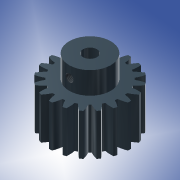
# Autodesk Inventor part: Spur Gear2
Saved by Autodesk Inventor 2017 SP1 (Build 210196100, 196)
## iProperties
Created: 2017-06-08
Part Number: Spur Gear2
Material: ABS Plastic
Document SubType Name: Modeling
Designer: zallen
Categories: <?xml version="1.0" encoding="UTF-16"?> <MemberInstance><Categories><FamilyTemplate><FamilyTemplateParameter ValueType="xs:double" Id="1" ObjectReferenceKey="da_z" ObjectType="kUserParameterObject"/><FamilyTemplateParameter ValueType="xs:double" Id="2" ObjectReferenceKey="da_b" ObjectType="kUserParameterObject"/><FamilyTemplateParameter ValueType="xs:double" Id="3" ObjectReferenceKey="da_beta" ObjectType="kUserParameterObject"/><FamilyTemplateParameter ValueType="xs:double" Id="4" ObjectReferenceKey="da_da" ObjectType="kUserParameterObject"/><FamilyTemplateParameter ValueType="xs:double" Id="5" ObjectReferenceKey="da_aw" ObjectType="kUserParameterObject"/><FamilyTemplateParameter ValueType="xs:string" Id="6" ObjectReferenceKey="EAIAABAAAACIAQAAAAAAAIAAAAAAAAAA" ObjectType="83910656" SubObjectId="SurfaceGeometry"/></FamilyTemplate><ParamToTemplateMap><ParamToTemplate CategoryParameter="//CategoryParameter[@InternalName='046C89C9-8512-4d59-83FE-43B91F4F132A']" TemplateParameter="1"/><ParamToTemplate CategoryParameter="//CategoryParameter[@InternalName='2552DF32-E462-4b46-AEBF-C6C7768E72AC']" TemplateParameter="2"/><ParamToTemplate CategoryParameter="//CategoryParameter[@InternalName='C9EE641D-15FC-4fae-A226-E94C4372FDD7']" TemplateParameter="3"/><ParamToTemplate><ParamToTemplate CategoryParameter="//CategoryParameter[@InternalName='00B6519A-459B-49c7-AD84-2E56D39A5744']" ConstantValue="0.000000"/></ParamToTemplate><ParamToTemplate><ParamToTemplate CategoryParameter="//CategoryParameter[@InternalName='04B31F0E-C7A6-4894-AA32-9629BEFACF47']" ConstantValue="1.000000"/></ParamToTemplate><ParamToTemplate><ParamToTemplate CategoryParameter="//CategoryParameter[@InternalName='43CBEC2E-7847-49e7-A936-2F7889FCB2D9']" ConstantValue="0.250000"/></ParamToTemplate><ParamToTemplate><ParamToTemplate CategoryParameter="//CategoryParameter[@InternalName='B1EFC894-105D-4ebd-86BF-FA20ED196853']" ConstantValue="0.350000"/></ParamToTemplate><ParamToTemplate><ParamToTemplate CategoryParameter="//CategoryParameter[@InternalName='51175063-3D10-4879-93E8-6246FE8B403D']" ConstantValue="2060000000.000000"/></ParamToTemplate><ParamToTemplate><ParamToTemplate CategoryParameter="//CategoryParameter[@InternalName='A3A52E27-4454-46a9-B0BD-C932399B70AF']" ConstantValue="0.300000"/></ParamToTemplate><ParamToTemplate><ParamToTemplate CategoryParameter="//CategoryParameter[@InternalName='91B76062-C214-41d9-B1B9-14D2AB99603D']" ConstantValue="0.130000"/></ParamToTemplate><ParamToTemplate><ParamToTemplate CategoryParameter="//CategoryParameter[@InternalName='374E806E-8B8A-4dda-A9AA-1039D6500AD2']" ConstantValue="7.692308"/></ParamToTemplate><ParamToTemplate><ParamToTemplate CategoryParameter="//CategoryParameter[@InternalName='2D373A89-B862-43d6-8D0B-0CBF12AB9F6C']" ConstantValue="0.349066"/></ParamToTemplate><ParamToTemplate CategoryParameter="//CategoryParameter[@InternalName='37777632-D6A2-4fac-9D53-DB8ACD95C989']" TemplateParameter="4"/><ParamToTemplate CategoryParameter="//CategoryParameter[@InternalName='FD1017F1-B727-4f7e-9707-0F86F1FF9423']" TemplateParameter="5"/><ParamToTemplate><ParamToTemplate CategoryParameter="//CategoryParameter[@InternalName='9E1B4470-B2D3-4ff1-B813-535BB4CDF51A']" ConstantValue="3520000.000000"/></ParamToTemplate><ParamToTemplate><ParamToTemplate CategoryParameter="//CategoryParameter[@InternalName='F8452263-BFF6-458c-9FB1-07C4B99E95CD']" ConstantValue="11400000.000000"/></ParamToTemplate><ParamToTemplate><ParamToTemplate CategoryParameter="//CategoryParameter[@InternalName='3E3BB259-FD49-497f-8171-6EBC954A3479']" ConstantValue="2.000000"/></ParamToTemplate><ParamToTemplate CategoryParameter="//CategoryParameter[@InternalName='27C3BAF2-7550-4e4b-AE2C-0DB134B7D9B7']" TemplateParameter="6"/></ParamToTemplateMap><Category DisplayName="Gear" InternalName="DC85795E-93AB-48d5-8EEE-5A27447B64BD" Mnemonic="Gear"><CategoryParameter DisplayName="z" InternalName="046C89C9-8512-4d59-83FE-43B91F4F132A" Mnemonic="z"/><CategoryParameter DisplayName="b" InternalName="2552DF32-E462-4b46-AEBF-C6C7768E72AC" Mnemonic="b"/><CategoryParameter DisplayName="||b|" InternalName="C9EE641D-15FC-4fae-A226-E94C4372FDD7" Mnemonic="beta"/><CategoryParameter DisplayName="x" InternalName="00B6519A-459B-49c7-AD84-2E56D39A5744" Mnemonic="x"/><CategoryParameter DisplayName="a*" InternalName="04B31F0E-C7A6-4894-AA32-9629BEFACF47" Mnemonic="a"/><CategoryParameter DisplayName="c*" InternalName="43CBEC2E-7847-49e7-A936-2F7889FCB2D9" Mnemonic="c"/><CategoryParameter DisplayName="r|.f|*" InternalName="B1EFC894-105D-4ebd-86BF-FA20ED196853" Mnemonic="rf"/><CategoryParameter DisplayName="E" InternalName="51175063-3D10-4879-93E8-6246FE8B403D" Mnemonic="E"/><CategoryParameter DisplayName="||m|" InternalName="A3A52E27-4454-46a9-B0BD-C932399B70AF" Mnemonic="mi"/><Category DisplayName="SpurGear" InternalName="26C5A22E-A91E-4dfd-A3B3-23CCAFAE1764" Mnemonic="SpurGear"><CategoryParameter DisplayName="m" InternalName="91B76062-C214-41d9-B1B9-14D2AB99603D" Mnemonic="m"/><CategoryParameter DisplayName="P" InternalName="374E806E-8B8A-4dda-A9AA-1039D6500AD2" Mnemonic="PP"/><CategoryParameter DisplayName="||a|" InternalName="2D373A89-B862-43d6-8D0B-0CBF12AB9F6C" Mnemonic="alpha"/><CategoryParameter DisplayName="d|.a|" InternalName="37777632-D6A2-4fac-9D53-DB8ACD95C989" Mnemonic="da"/><CategoryParameter DisplayName="a|.w|" InternalName="FD1017F1-B727-4f7e-9707-0F86F1FF9423" Mnemonic="aw"/><CategoryParameter DisplayName="||s||.Flim|" InternalName="9E1B4470-B2D3-4ff1-B813-535BB4CDF51A" Mnemonic="sFlim"/><CategoryParameter DisplayName="||s||.Hlim|" InternalName="F8452263-BFF6-458c-9FB1-07C4B99E95CD" Mnemonic="sHlim"/><CategoryParameter DisplayName="type" InternalName="3E3BB259-FD49-497f-8171-6EBC954A3479" Mnemonic="type"/><CategoryParameter DisplayName="PitchDiameter" InternalName="27C3BAF2-7550-4e4b-AE2C-0DB134B7D9B7" Mnemonic="IDS_PITCHDIAM"/></Category></Category></Categories></MemberInstance>
Density: 1.06 g/cm^3
Appearance: CR Dark Blue
CustomPartVersion: 1
Author: zallen
Autodesk Inventor part; units mm, degrees
sketch "Sketch1" plane through (0, 0, 0) normal (0, 0, 1) x (1, 0, 0)
  circle A0 centre (0, 0) radius 14.3
  dimension "d0" = 28.6
  constraints: 1 centre point
  measures "d0" diameter of A0
extrude "Extrusion1" add sketch "Sketch1" along normal blind 15
ref_plane "Work Plane2" through (0, 0, 7.5) normal (0, 0, 1) x (1, 0, 0)
sketch "Sketch2" plane through (0, 0, 0) normal (0, 0, -1) x (-1, 0, 0)
  circle A0 centre (0, 0) radius 14.3 projected
  circle A1 centre (0, 0) radius 13
  dimension "d3" = 26
  constraints: 1 centre point, 1 coincident
  measures "d3" diameter of A1
surface extrude "Pitch Diameter" sketch "Sketch2" against normal through all shown no curves A1
ref_plane "Work Plane8" through (0, 0, 0) normal (0.9876883, 0.1564345, 0) x (0, 0, 1)
ref_plane "Work Plane9" through (0, 0, 0) normal (1, 0, 0) x (0, 1, 0)
spur gear teeth "Spur Gear" teeth 20 pitch diameter 26 tip diameter 28.6 root diameter 22.75 face width 15 start plane through (0, 0, 0) normal (0, 0, -1) x (-1, 0, 0)
sketch "Sketch3" plane through (0, 0, 15) normal (0, 0, 1) x (1, 0, 0)
  circle A0 centre (0, 0) radius 2.5
  dimension "d49" = 5
  constraints: 1 centre point, 1 coincident
  measures "d49" diameter of A0
extrude "Extrusion2" cut sketch "Sketch3" against normal through all
sketch "Sketch4" plane through (0, 0, 15) normal (0, 0, 1) x (1, 0, 0)
  circle A0 centre (0, 0) radius 7.5
  circle A1 centre (0, 0) radius 2.5
  circle A2 centre (0, 0) radius 2.5 projected
  arc A3 (-4.9495, 13.4161) -> (-4.7623, 10.3301) centre (5.7891, 12.5189) ccw projected
  arc A4 (-4.7623, 10.3301) -> (-5.5581, 9.9246) centre (0, 0) ccw projected
  arc A5 (-5.5581, 9.9246) -> (-7.9447, 11.89) centre (-13.5308, 2.6749) ccw projected
  arc A6 (-7.9447, 11.89) -> (-8.853, 11.23) centre (0, 0) ccw projected
  arc A7 (-8.853, 11.23) -> (-7.7214, 8.3529) centre (1.6372, 13.6952) ccw projected
  arc A8 (-7.7214, 8.3529) -> (-8.3529, 7.7214) centre (0, 0) ccw projected
  arc A9 (-8.3529, 7.7214) -> (-11.23, 8.853) centre (-13.6952, -1.6372) ccw projected
  arc A10 (-11.23, 8.853) -> (-11.89, 7.9447) centre (0, 0) ccw projected
  arc A11 (-11.89, 7.9447) -> (-9.9246, 5.5581) centre (-2.6749, 13.5308) ccw projected
  arc A12 (-9.9246, 5.5581) -> (-10.3301, 4.7623) centre (0, 0) ccw projected
  arc A13 (-10.3301, 4.7623) -> (-13.4161, 4.9495) centre (-12.5189, -5.7891) ccw projected
  arc A14 (-13.4161, 4.9495) -> (-13.7631, 3.8816) centre (0, 0) ccw projected
  arc A15 (-13.7631, 3.8816) -> (-11.1564, 2.2192) centre (-6.7253, 12.042) ccw projected
  arc A16 (-11.1564, 2.2192) -> (-11.2962, 1.337) centre (0, 0) ccw projected
  arc A17 (-11.2962, 1.337) -> (-14.289, 0.5614) centre (-10.1173, -9.3744) ccw projected
  arc A18 (-14.289, 0.5614) -> (-14.289, -0.5614) centre (0, 0) ccw projected
  arc A19 (-14.289, -0.5614) -> (-11.2962, -1.337) centre (-10.1173, 9.3744) ccw projected
  arc A20 (-11.2962, -1.337) -> (-11.1564, -2.2192) centre (0, 0) ccw projected
  arc A21 (-11.1564, -2.2192) -> (-13.7631, -3.8816) centre (-6.7253, -12.042) ccw projected
  arc A22 (-13.7631, -3.8816) -> (-13.4161, -4.9495) centre (0, 0) ccw projected
  arc A23 (-13.4161, -4.9495) -> (-10.3301, -4.7623) centre (-12.5189, 5.7891) ccw projected
  arc A24 (-10.3301, -4.7623) -> (-9.9246, -5.5581) centre (0, 0) ccw projected
  arc A25 (-9.9246, -5.5581) -> (-11.89, -7.9447) centre (-2.6749, -13.5308) ccw projected
  arc A26 (-11.89, -7.9447) -> (-11.23, -8.853) centre (0, 0) ccw projected
  arc A27 (-11.23, -8.853) -> (-8.3529, -7.7214) centre (-13.6952, 1.6372) ccw projected
  arc A28 (-8.3529, -7.7214) -> (-7.7214, -8.3529) centre (0, 0) ccw projected
  arc A29 (-7.7214, -8.3529) -> (-8.853, -11.23) centre (1.6372, -13.6952) ccw projected
  arc A30 (-8.853, -11.23) -> (-7.9447, -11.89) centre (0, 0) ccw projected
  arc A31 (-7.9447, -11.89) -> (-5.5581, -9.9246) centre (-13.5308, -2.6749) ccw projected
  arc A32 (-5.5581, -9.9246) -> (-4.7623, -10.3301) centre (0, 0) ccw projected
  arc A33 (-4.7623, -10.3301) -> (-4.9495, -13.4161) centre (5.7891, -12.5189) ccw projected
  arc A34 (-4.9495, -13.4161) -> (-3.8816, -13.7631) centre (0, 0) ccw projected
  arc A35 (-3.8816, -13.7631) -> (-2.2192, -11.1564) centre (-12.042, -6.7253) ccw projected
  arc A36 (-2.2192, -11.1564) -> (-1.337, -11.2962) centre (0, 0) ccw projected
  arc A37 (-1.337, -11.2962) -> (-0.5614, -14.289) centre (9.3744, -10.1173) ccw projected
  arc A38 (-0.5614, -14.289) -> (0.5614, -14.289) centre (0, 0) ccw projected
  arc A39 (0.5614, -14.289) -> (1.337, -11.2962) centre (-9.3744, -10.1173) ccw projected
  arc A40 (1.337, -11.2962) -> (2.2192, -11.1564) centre (0, 0) ccw projected
  arc A41 (2.2192, -11.1564) -> (3.8816, -13.7631) centre (12.042, -6.7253) ccw projected
  arc A42 (3.8816, -13.7631) -> (4.9495, -13.4161) centre (0, 0) ccw projected
  arc A43 (4.9495, -13.4161) -> (4.7623, -10.3301) centre (-5.7891, -12.5189) ccw projected
  arc A44 (4.7623, -10.3301) -> (5.5581, -9.9246) centre (0, 0) ccw projected
  arc A45 (5.5581, -9.9246) -> (7.9447, -11.89) centre (13.5308, -2.6749) ccw projected
  arc A46 (7.9447, -11.89) -> (8.853, -11.23) centre (0, 0) ccw projected
  arc A47 (8.853, -11.23) -> (7.7214, -8.3529) centre (-1.6372, -13.6952) ccw projected
  arc A48 (7.7214, -8.3529) -> (8.3529, -7.7214) centre (0, 0) ccw projected
  arc A49 (8.3529, -7.7214) -> (11.23, -8.853) centre (13.6952, 1.6372) ccw projected
  arc A50 (11.23, -8.853) -> (11.89, -7.9447) centre (0, 0) ccw projected
  arc A51 (11.89, -7.9447) -> (9.9246, -5.5581) centre (2.6749, -13.5308) ccw projected
  arc A52 (9.9246, -5.5581) -> (10.3301, -4.7623) centre (0, 0) ccw projected
  arc A53 (10.3301, -4.7623) -> (13.4161, -4.9495) centre (12.5189, 5.7891) ccw projected
  arc A54 (13.4161, -4.9495) -> (13.7631, -3.8816) centre (0, 0) ccw projected
  arc A55 (13.7631, -3.8816) -> (11.1564, -2.2192) centre (6.7253, -12.042) ccw projected
  arc A56 (11.1564, -2.2192) -> (11.2962, -1.337) centre (0, 0) ccw projected
  arc A57 (11.2962, -1.337) -> (14.289, -0.5614) centre (10.1173, 9.3744) ccw projected
  arc A58 (14.289, -0.5614) -> (14.289, 0.5614) centre (0, 0) ccw projected
  arc A59 (14.289, 0.5614) -> (11.2962, 1.337) centre (10.1173, -9.3744) ccw projected
  arc A60 (11.2962, 1.337) -> (11.1564, 2.2192) centre (0, 0) ccw projected
  arc A61 (11.1564, 2.2192) -> (13.7631, 3.8816) centre (6.7253, 12.042) ccw projected
  arc A62 (13.7631, 3.8816) -> (13.4161, 4.9495) centre (0, 0) ccw projected
  arc A63 (13.4161, 4.9495) -> (10.3301, 4.7623) centre (12.5189, -5.7891) ccw projected
  arc A64 (10.3301, 4.7623) -> (9.9246, 5.5581) centre (0, 0) ccw projected
  arc A65 (9.9246, 5.5581) -> (11.89, 7.9447) centre (2.6749, 13.5308) ccw projected
  arc A66 (11.89, 7.9447) -> (11.23, 8.853) centre (0, 0) ccw projected
  arc A67 (11.23, 8.853) -> (8.3529, 7.7214) centre (13.6952, -1.6372) ccw projected
  arc A68 (8.3529, 7.7214) -> (7.7214, 8.3529) centre (0, 0) ccw projected
  arc A69 (7.7214, 8.3529) -> (8.853, 11.23) centre (-1.6372, 13.6952) ccw projected
  arc A70 (8.853, 11.23) -> (7.9447, 11.89) centre (0, 0) ccw projected
  arc A71 (7.9447, 11.89) -> (5.5581, 9.9246) centre (13.5308, 2.6749) ccw projected
  arc A72 (5.5581, 9.9246) -> (4.7623, 10.3301) centre (0, 0) ccw projected
  arc A73 (4.7623, 10.3301) -> (4.9495, 13.4161) centre (-5.7891, 12.5189) ccw projected
  arc A74 (4.9495, 13.4161) -> (3.8816, 13.7631) centre (0, 0) ccw projected
  arc A75 (3.8816, 13.7631) -> (2.2192, 11.1564) centre (12.042, 6.7253) ccw projected
  arc A76 (2.2192, 11.1564) -> (1.337, 11.2962) centre (0, 0) ccw projected
  arc A77 (1.337, 11.2962) -> (0.5614, 14.289) centre (-9.3744, 10.1173) ccw projected
  arc A78 (0.5614, 14.289) -> (-0.5614, 14.289) centre (0, 0) ccw projected
  arc A79 (-0.5614, 14.289) -> (-1.337, 11.2962) centre (9.3744, 10.1173) ccw projected
  arc A80 (-1.337, 11.2962) -> (-2.2192, 11.1564) centre (0, 0) ccw projected
  arc A81 (-2.2192, 11.1564) -> (-3.8816, 13.7631) centre (-12.042, 6.7253) ccw projected
  arc A82 (-3.8816, 13.7631) -> (-4.9495, 13.4161) centre (0, 0) ccw projected
  dimension "d52" = 15
  constraints: 2 centre point, 2 coincident, 1 concentric
  measures "d52" diameter of A0
extrude "Extrusion3" add sketch "Sketch4" along normal blind 8 contours A0
sketch "Sketch5" plane through (0, 0, 0) normal (0, 1, 0) x (-1, 0, 0)
  circle A0 centre (0, 19) radius 1.4
  line L0 (7.5, 15) -> (7.5, 23) projected
  point P0 (0, 0)
  point P1 (7.5, 19)
  dimension "d55" = 2.8
  constraints: 1 centre point, 1 horizontal alignment, 1 midpoint, 1 vertical alignment
  measures "d55" diameter of A0
extrude "Extrusion4" cut sketch "Sketch5" against normal through all
thread "Thread1" size "M3x0.5" class "6H" standard "ANSI Metric M Profile" full length
equation "\"d0\" = da_da"
equation "\"d1\" = da_b"
equation "\"d3\" = da_dw"
equation "\"d16\" = da_aw"
equation "\"d43\" = da_aw"
equation "\"d46\" = da_aw"
equation "\"da_da\" = 28.6"
equation "\"da_b\" = 15"
equation "\"da_dw\" = 26"
equation "\"da_aw\" = 65"
body "Solid1"
body "Srf1"
